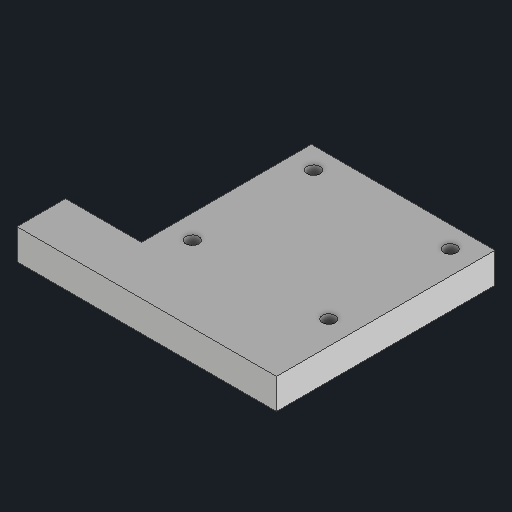
# Autodesk Inventor part: Seiten_Platte
Saved by Autodesk Inventor 2026 (Build 300175000, 175)
## iProperties
Created: 2025-09-01
Part Number: Seiten_Platte
Material: Generisch
Document SubType Name: Modeling
Designer: weyer
Density: 1 g/cm^3
Appearance: Vorgabe
Author: weyer
Autodesk Inventor part; units mm, degrees
ref_plane "YZ Plane" through (0, 0, 0) normal (1, 0, 0) x (0, 1, 0)
ref_plane "XZ Plane" through (0, 0, 0) normal (0, 1, 0) x (-1, 0, 0)
ref_plane "XY Plane" through (0, 0, 0) normal (0, 0, 1) x (1, 0, 0)
sketch "Skizze1" plane through (0, 0, 0) normal (0, 0, 1) x (1, 0, 0)
  circle A0 centre (17.75, 57) radius 2.15 projected
  circle A1 centre (62.75, 57) radius 2.15 projected
  circle A2 centre (17.75, 17) radius 2.15 projected
  circle A3 centre (62.75, 17) radius 2.15 projected
  line L0 (70.5, 64) -> (10, 64) projected
  line L1 (10, 64) -> (10, -3) projected
  line L2 (70.5, -3) -> (70.5, 64) projected
  line L3 (10, -3) -> (70.5, -3) projected
  line L4 (0, 0) -> (0, 8) projected
  line L5 (0, 8) -> (-15, 8) projected
  line L6 (-15, -8) -> (-15, 8) projected
  line L7 (0, -8) -> (-15, -8) projected
  line L8 (70.5, -8) -> (70.5, 64)
  line L9 (10, 64) -> (10, 8)
  line L10 (-15, 8) -> (10, 8)
  line L11 (70.5, -8) -> (-15, -8)
  line L12 (-15, 8) -> (-15, -8)
  point P0 (-10, 0)
  dimension "d0" = 16
  constraints: 10 end point, 2 point on line, 1 collinear, 1 horizontal, 1 parallel, 1 perpendicular, 1 other
  measures "d0" distance of L5.end L11.end
extrude "Extrusion1" add sketch "Skizze1" along normal blind 10
